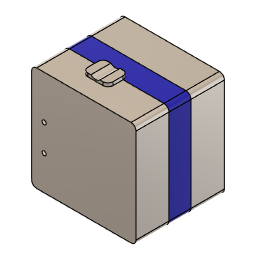
OpenBCI_ESP v18 (Autodesk Fusion 360 design; units mm, degrees)
Autodesk Fusion 360 part; units mm, degrees
sketch "Sketch1" plane through (0, 0, 0) normal (0, 0, 1) x (1, 0, 0)
  line L0 (0, 0) -> (62.5, 0)
  line L1 (62.5, 0) -> (62.5, 62.5)
  line L2 (62.5, 62.5) -> (0, 62.5)
  line L3 (0, 62.5) -> (0, 0)
  line L4 (60, 53.4185) -> (60.5, 53.4185)
  line L5 (60, 6.9185) -> (60.5, 6.9185)
  line L6 (2.5, 53.4185) -> (2, 53.4185)
  circle A0 centre (4.5, 58) radius 1.1
  circle A1 centre (58, 58) radius 1.1
  circle A2 centre (58, 4.5) radius 1.1
  circle A3 centre (4.5, 4.5) radius 1.1
  line L7 (0, 55.25) -> (62.5, 55.25)
  line L8 (0, 7.25) -> (62.5, 7.25)
  line L9 (1.75, 55.25) -> (1.75, 7.25)
  line L10 (60.75, 55.25) -> (60.75, 7.25)
  line L11 (7, 55.25) -> (55.5, 55.25)
  line L12 (55.5, 55.25) -> (55.5, 60)
  line L13 (55.5, 60) -> (7, 60)
  line L14 (7, 60) -> (7, 55.25)
  line L15 (7, 7.25) -> (55.5, 7.25)
  line L16 (55.5, 7.25) -> (55.5, 2.5)
  line L17 (55.5, 2.5) -> (7, 2.5)
  line L18 (7, 2.5) -> (7, 7.25)
  line L19 (10, 60) -> (13.3303, 60)
  line L20 (13.3303, 60) -> (13.3303, 56.25)
  line L21 (13.3303, 56.25) -> (10, 56.25)
  line L22 (10, 56.25) -> (10, 60)
  line L23 (10, 7.25) -> (13.75, 7.25)
  line L24 (13.75, 7.25) -> (13.75, 2.5)
  line L25 (13.75, 2.5) -> (10, 2.5)
  line L26 (10, 2.5) -> (10, 7.25)
  line L27 (40.75, 60) -> (44.5, 60)
  line L28 (44.5, 60) -> (44.5, 56.25)
  line L29 (44.5, 56.25) -> (40.75, 56.25)
  line L30 (40.75, 56.25) -> (40.75, 60)
  line L31 (40.75, 7.25) -> (44.5, 7.25)
  line L32 (44.5, 7.25) -> (44.5, 2.5)
  line L33 (44.5, 2.5) -> (40.75, 2.5)
  line L34 (40.75, 2.5) -> (40.75, 7.25)
  circle A4 centre (4.5, 58) radius 1.9
  circle A5 centre (58, 58) radius 1.9
  circle A6 centre (4.5, 4.5) radius 1.9
  circle A7 centre (58, 4.5) radius 1.9
  line L35 (10, 6.25) -> (13.75, 6.25)
  line L36 (40.75, 6.25) -> (44.5, 6.25)
  dimension "d1" = 62.5
  dimension "d2" = 62.5
  dimension "d5" = 57.5
  dimension "d8" = 2.2
  dimension "d9" = 4.5
  dimension "d10" = 4.5
  dimension "d11" = 2.2
  dimension "d12" = 4.5
  dimension "d13" = 4.5
  dimension "d14" = 2.2
  dimension "d15" = 4.5
  dimension "d16" = 4.5
  dimension "d17" = 2.2
  dimension "d18" = 4.5
  dimension "d19" = 4.5
  dimension "d25" = 7.25
  dimension "d26" = 7.25
  dimension "d27" = 48
  dimension "d28" = 1.75
  dimension "d29" = 1.75
  dimension "d30" = 59
  dimension "d34" = 2.5
  dimension "d35" = 7
  dimension "d36" = 7
  dimension "d37" = 7
  dimension "d38" = 7
  dimension "d39" = 2.5
  dimension "d201" = 3.75
  dimension "d202" = 10
  dimension "d203" = 3.75
  dimension "d204" = 10
  dimension "d205" = 3.75
  dimension "d206" = 18
  dimension "d207" = 3.75
  dimension "d208" = 18
  dimension "d215" = 3.8
  dimension "d216" = 3.8
  dimension "d217" = 3.8
  dimension "d218" = 3.8
  dimension "d219" = 3.75
  dimension "d220" = 3.75
  constraint horizontal L0
  constraint vertical L1
  constraint horizontal L2
  constraint vertical L3
  constraint coincident L0.start L3.end
  constraint coincident L3 L7.start
  constraint coincident L1 L7.end
  constraint perpendicular L1 L7
  constraint coincident L3 L8.start
  constraint coincident L1 L8.end
  constraint perpendicular L1 L8
  constraint coincident L7 L9.start
  constraint coincident L8 L9.end
  constraint perpendicular L8 L9
  constraint coincident L7 L10.start
  constraint coincident L8 L10.end
  constraint perpendicular L8 L10
  constraint horizontal L11
  constraint vertical L12
  constraint horizontal L13
  constraint vertical L14
  constraint coincident L7 L11.start
  constraint horizontal L15
  constraint vertical L16
  constraint horizontal L17
  constraint vertical L18
  constraint coincident L8 L15.start
  constraint horizontal L19
  constraint vertical L20
  constraint horizontal L21
  constraint vertical L22
  constraint coincident L13 L19.start
  constraint horizontal L23
  constraint vertical L24
  constraint horizontal L25
  constraint vertical L26
  constraint coincident L15 L23.start
  constraint horizontal L27
  constraint vertical L28
  constraint horizontal L29
  constraint vertical L30
  constraint coincident L13 L27.start
  constraint horizontal L31
  constraint vertical L32
  constraint horizontal L33
  constraint vertical L34
  constraint coincident L8 L31.start
  constraint concentric A0 A4
  constraint concentric A1 A5
  constraint concentric A3 A6
  constraint concentric A2 A7
  constraint coincident L26 L35.start
  constraint coincident L24 L35.end
  constraint perpendicular L24 L35
  constraint coincident L34 L36.start
  constraint coincident L32 L36.end
  constraint perpendicular L32 L36
  measures "d1" distance of L0.start L0.end
  measures "d2" distance of L0.start L2.end
  measures "d5" distance of L6.start L4.start
  measures "d8" diameter of A0
  measures "d9" distance of L3 A0.centre
  measures "d10" distance of L2 A0.centre
  measures "d11" diameter of A1
  measures "d12" distance of L1 A1.centre
  measures "d13" distance of L2 A1.centre
  measures "d14" diameter of A2
  measures "d15" distance of L1 A2.centre
  measures "d16" distance of L0 A2.centre
  measures "d17" diameter of A3
  measures "d18" distance of L3 A3.centre
  measures "d19" distance of L0 A3.centre
  measures "d25" distance of L2 L7
  measures "d26" distance of L0 L8
  measures "d27" distance of L7 L8
  measures "d28" distance of L1 L10
  measures "d29" distance of L3 L9
  measures "d30" distance of L9 L10
  measures "d34" distance of L2 L13
  measures "d35" distance of L1 L12
  measures "d36" distance of L3 L14
  measures "d37" distance of L1 L16
  measures "d38" distance of L3 L18
  measures "d39" distance of L0 L17
  measures "d201" distance of L19.start L21.end
  measures "d202" distance of L3 L22
  measures "d203" distance of L23.start L23.end
  measures "d204" distance of L3 L26
  measures "d205" distance of L27.start L27.end
  measures "d206" distance of L1 L28
  measures "d207" distance of L31.start L31.end
  measures "d208" distance of L1 L32
  measures "d215" diameter of A4
  measures "d216" diameter of A5
  measures "d217" diameter of A6
  measures "d218" diameter of A7
  measures "d219" distance of L17 L35
  measures "d220" distance of L17 L36
extrude "Extrude1" add sketch "Sketch1" along normal blind 2 contours L0 L1 L3 L8 L16 L17 L18 L25 L33 | L3 L7 L8 L9 | L1 L7 L8 L10 | L1 L2 L3 L7 L12 L13 L14 L19 L27 | L7 L8 L9 L10 L11 L15 L23 L31 | L8 L15 L17 L18 L26 | L8 L15 L16 L17 L32 | L7 L11 L12 L13 L14 L20 L21 L22 L28 L29 L30 | L8 L15 L23 L24 L26 L35 | L8 L15 L31 L32 L34 L36 | L8 L15 L17 L24 L34 | L17 L24 L25 L26 L35 | L17 L32 L33 L34 L36 | L13 L19 L20 L21 L22 | L13 L27 L28 L29 L30 | A4 | A5 | A6 | A7 makes body 1
extrude "Extrude2" add sketch "Sketch1" along normal blind 20 contours L0 L1 L3 L8 L16 L17 L18 L25 L33 | L3 L7 L8 L9 | L1 L7 L8 L10 | L1 L2 L3 L7 L12 L13 L14 L19 L27 | A4 | A5 | A6 | A7 bodies 1
extrude "Extrude18" add sketch "Sketch1" along normal blind 10 from surface at 15 contours L17 L24 L25 L26 L35 | L17 L32 L33 L34 L36 | L13 L19 L20 L21 L22 | L13 L27 L28 L29 L30 bodies 1
chamfer "Chamfer3" distance 3.5 angle 45 4 edges at (11.6651, 56.25, 15) (42.625, 56.25, 15) (42.625, 6.25, 15) (11.875, 6.25, 15) on bodies 1
fillet "Fillet7" radius 3 4 edges at (0, 62.5, 10) (0, 0, 10) (62.5, 62.5, 10) (62.5, 0, 10) on bodies 1
extrude "Extrude20" cut sketch "Sketch1" along normal blind 9 contours A4 | A5 | A6 | A7 bodies 1
sketch "Sketch2" plane through (0, 0, 20) normal (0, 0, 1) x (1, 0, 0)
  line L0 (0, 0) -> (62.5, 0)
  line L1 (62.5, 0) -> (62.5, 62.5)
  line L2 (62.5, 62.5) -> (0, 62.5)
  line L3 (0, 62.5) -> (0, 0)
  line L4 (2, 56.5) -> (52.5, 56.5)
  line L5 (52.5, 56.5) -> (52.5, 6)
  line L6 (52.5, 6) -> (2, 6)
  line L7 (2, 6) -> (2, 56.5)
  circle A0 centre (6, 52.9441) radius 1.1
  circle A1 centre (48.5, 52.5) radius 1.1
  circle A2 centre (6, 10) radius 1.1
  circle A3 centre (48.5, 10) radius 1.1
  line L8 (2, 56.5) -> (10, 56.5)
  line L9 (10, 56.5) -> (10, 48.5)
  line L10 (10, 48.5) -> (2, 48.5)
  line L11 (2, 48.5) -> (2, 56.5)
  line L12 (2, 6) -> (10, 6)
  line L13 (10, 6) -> (10, 14)
  line L14 (10, 14) -> (2, 14)
  line L15 (2, 14) -> (2, 6)
  line L16 (52.5, 6) -> (44.5, 6)
  line L17 (44.5, 6) -> (44.5, 14)
  line L18 (44.5, 14) -> (52.5, 14)
  line L19 (52.5, 14) -> (52.5, 6)
  line L20 (52.5, 56.5) -> (44.5, 56.5)
  line L21 (44.5, 56.5) -> (44.5, 48.5)
  line L22 (44.5, 48.5) -> (52.5, 48.5)
  line L23 (52.5, 48.5) -> (52.5, 56.5)
  line L24 (2, 46.25) -> (0, 46.25)
  line L25 (2, 16.25) -> (0, 16.25)
  line L26 (52.5, 48.5) -> (59.5, 48.5)
  line L27 (59.5, 48.5) -> (59.5, 14)
  line L28 (59.5, 14) -> (52.5, 14)
  line L29 (52.5, 14) -> (52.5, 48.5)
  line L30 (10, 6) -> (44.5, 6)
  line L31 (44.5, 6) -> (44.5, 2.5)
  line L32 (44.5, 2.5) -> (10, 2.5)
  line L33 (10, 2.5) -> (10, 6)
  line L34 (10, 56.5) -> (44.5, 56.5)
  line L35 (44.5, 56.5) -> (44.5, 60)
  line L36 (44.5, 60) -> (10, 60)
  line L37 (10, 60) -> (10, 56.5)
  circle A4 centre (6, 52.9441) radius 0.9
  circle A5 centre (48.5, 52.5) radius 0.9
  circle A6 centre (48.5, 10) radius 0.9
  circle A7 centre (6, 10) radius 0.9
  circle A8 centre (7.5, 36.5) radius 1.25
  circle A9 centre (7.5, 20.5) radius 1.25
  circle A10 centre (18, 36.5) radius 1.25
  circle A11 centre (4.5, 58) radius 0.9
  circle A12 centre (4.5, 4.5) radius 0.9
  circle A13 centre (58, 4.5) radius 0.9
  circle A14 centre (58, 58) radius 0.9
  line L38 (44.5, 60) -> (39.5, 60)
  line L39 (39.5, 56.5) -> (44.5, 56.5)
  line L40 (44.5, 56.5) -> (44.5, 60)
  line L41 (10, 60) -> (15, 60)
  line L42 (15, 60) -> (15, 56.5)
  line L43 (15, 56.5) -> (10, 56.5)
  line L44 (10, 56.5) -> (10, 60)
  line L45 (44.5, 2.5) -> (39.5, 2.5)
  line L46 (39.5, 6) -> (44.5, 6)
  line L47 (44.5, 6) -> (44.5, 2.5)
  line L48 (10, 2.5) -> (15, 2.5)
  line L49 (15, 2.5) -> (15, 6)
  line L50 (15, 6) -> (10, 6)
  line L51 (10, 6) -> (10, 2.5)
  line L52 (59.5, 48.5) -> (56, 48.5)
  line L53 (56, 48.5) -> (56, 43.5)
  line L54 (56, 43.5) -> (59.5, 43.5)
  line L55 (59.5, 43.5) -> (59.5, 48.5)
  line L56 (59.5, 14) -> (56, 14)
  line L57 (56, 14) -> (56, 19)
  line L58 (56, 19) -> (59.5, 19)
  line L59 (59.5, 19) -> (59.5, 14)
  dimension "d42" = 62.5
  dimension "d43" = 62.5
  dimension "d44" = 50.5
  dimension "d45" = 50.5
  dimension "d46" = 6
  dimension "d47" = 2
  dimension "d48" = 2.2
  dimension "d49" = 4
  dimension "d50" = 2.2
  dimension "d51" = 4
  dimension "d52" = 4
  dimension "d53" = 2.2
  dimension "d54" = 2.2
  dimension "d55" = 4
  dimension "d56" = 4
  dimension "d57" = 4
  dimension "d58" = 4
  dimension "d59" = 8
  dimension "d60" = 8
  dimension "d61" = 8
  dimension "d62" = 8
  dimension "d63" = 8
  dimension "d64" = 8
  dimension "d65" = 8
  dimension "d66" = 8
  dimension "d67" = 30
  dimension "d68" = 10.25
  dimension "d69" = 7
  dimension "d70" = 3.5
  dimension "d71" = 3.5
  dimension "d105" = 1.8
  dimension "d106" = 1.8
  dimension "d107" = 1.8
  dimension "d108" = 1.8
  dimension "d109" = 2.5
  dimension "d110" = 2.5
  dimension "d111" = 2.5
  dimension "d112" = 5.5
  dimension "d113" = 5.5
  dimension "d114" = 14.5
  dimension "d115" = 20
  dimension "d116" = 20
  dimension "d117" = 16
  dimension "d133" = 1.8
  dimension "d135" = 1.8
  dimension "d136" = 1.8
  dimension "d137" = 4.5
  dimension "d138" = 4.5
  dimension "d139" = 4.5
  dimension "d140" = 4.5
  dimension "d141" = 4.5
  dimension "d142" = 4.5
  dimension "d145" = 1.8
  dimension "d146" = 4.5
  dimension "d147" = 4.5
  dimension "d176" = 16
  dimension "d189" = 3.5
  dimension "d190" = 5
  dimension "d191" = 3.5
  dimension "d193" = 3.5
  dimension "d194" = 5
  dimension "d195" = 3.5
  dimension "d223" = 3.5
  dimension "d224" = 5
  dimension "d225" = 3.5
  dimension "d226" = 5
  constraint horizontal L0
  constraint vertical L1
  constraint horizontal L2
  constraint vertical L3
  constraint coincident L0.start L3.end
  constraint horizontal L4
  constraint vertical L5
  constraint horizontal L6
  constraint vertical L7
  constraint horizontal L8
  constraint vertical L9
  constraint horizontal L10
  constraint vertical L11
  constraint horizontal L12
  constraint vertical L13
  constraint horizontal L14
  constraint vertical L15
  constraint horizontal L16
  constraint vertical L17
  constraint horizontal L18
  constraint vertical L19
  constraint horizontal L20
  constraint vertical L21
  constraint horizontal L22
  constraint vertical L23
  constraint coincident L7 L24.start
  constraint coincident L3 L24.end
  constraint perpendicular L3 L24
  constraint coincident L7 L25.start
  constraint coincident L3 L25.end
  constraint perpendicular L7 L25
  constraint horizontal L26
  constraint vertical L27
  constraint horizontal L28
  constraint vertical L29
  constraint horizontal L30
  constraint vertical L31
  constraint horizontal L32
  constraint vertical L33
  constraint horizontal L34
  constraint vertical L35
  constraint horizontal L36
  constraint vertical L37
  constraint concentric A0 A4
  constraint concentric A1 A5
  constraint concentric A3 A6
  constraint concentric A2 A7
  constraint horizontal L38
  constraint horizontal L39
  constraint vertical L40
  constraint horizontal L41
  constraint vertical L42
  constraint horizontal L43
  constraint vertical L44
  constraint horizontal L45
  constraint horizontal L46
  constraint vertical L47
  constraint horizontal L48
  constraint vertical L49
  constraint horizontal L50
  constraint vertical L51
  constraint horizontal L52
  constraint vertical L53
  constraint horizontal L54
  constraint vertical L55
  constraint horizontal L56
  constraint vertical L57
  constraint horizontal L58
  constraint vertical L59
  measures "d42" distance of L1 L3
  measures "d43" distance of L0 L2
  measures "d44" distance of L4.start L4.end
  measures "d45" distance of L4.start L6.end
  measures "d46" distance of L2 L4
  measures "d47" distance of L3 L7
  measures "d48" diameter of A0
  measures "d49" distance of L7 A0.centre
  measures "d50" diameter of A1
  measures "d51" distance of L5 A1.centre
  measures "d52" distance of L4 A1.centre
  measures "d53" diameter of A2
  measures "d54" diameter of A3
  measures "d55" distance of L5 A3.centre
  measures "d56" distance of L6 A3.centre
  measures "d57" distance of L6 A2.centre
  measures "d58" distance of L7 A2.centre
  measures "d59" distance of L4.start L8.end
  measures "d60" distance of L4.start L10.end
  measures "d61" distance of L6.end L12.end
  measures "d62" distance of L6.end L14.end
  measures "d63" distance of L5.end L16.end
  measures "d64" distance of L5.end L18.end
  measures "d65" distance of L4.end L20.end
  measures "d66" distance of L4.end L22.end
  measures "d67" distance of L24 L25
  measures "d68" distance of L12 L25
  measures "d69" distance of L22.end L26.end
  measures "d70" distance of L12.end L32.end
  measures "d71" distance of L8.end L36.end
  measures "d105" diameter of A4
  measures "d106" diameter of A5
  measures "d107" diameter of A6
  measures "d108" diameter of A7
  measures "d109" diameter of A8
  measures "d110" diameter of A9
  measures "d111" diameter of A10
  measures "d112" distance of L7 A8.centre
  measures "d113" distance of L7 A9.centre
  measures "d114" distance of L30 A9.centre
  measures "d115" distance of L34 A8.centre
  measures "d116" distance of L4 A10.centre
  measures "d117" distance of L7 A10.centre
  measures "d133" diameter of A11
  measures "d135" diameter of A12
  measures "d136" diameter of A13
  measures "d137" distance of L1 A13.centre
  measures "d138" distance of L0 A13.centre
  measures "d139" distance of L3 A12.centre
  measures "d140" distance of L0 A12.centre
  measures "d141" distance of L3 A11.centre
  measures "d142" distance of L2 A11.centre
  measures "d145" diameter of A14
  measures "d146" distance of L2 A14.centre
  measures "d147" distance of L1 A14.centre
  measures "d176" distance of A8.centre A9.centre
  measures "d189" distance of L35.end L20.end
  measures "d190" distance of L36.end L41.end
  measures "d191" distance of L36.end L8.end
  measures "d193" distance of L31.end L16.end
  measures "d194" distance of L32.end L48.end
  measures "d195" distance of L32.end L12.end
  measures "d223" distance of L26.end L52.end
  measures "d224" distance of L26.end L54.end
  measures "d225" distance of L27.end L56.end
  measures "d226" distance of L27.end L58.end
extrude "Extrude3" add sketch "Sketch2" along normal blind 2 separate body contours L0 L1 L2 L3 L4 L5 L6 L7 L8 L11 L12 L15 L16 L19 L20 L23 L24 L25 L26 L27 L28 L31 L32 L33 L35 L36 L37 L38 L40 L41 L44 L45 L47 L48 L51 L52 L55 L56 L59 makes body 2
extrude "Extrude4" add sketch "Sketch2" along normal blind 11.2 from surface at 2 contours L0 L1 L2 L3 L4 L5 L6 L7 L8 L11 L12 L15 L16 L19 L20 L23 L24 L25 L26 L27 L28 L31 L32 L33 L35 L36 L37 L38 L40 L41 L44 L45 L47 L48 L51 L52 L55 L56 L59 | L6 L7 L12 L13 L14 L15 | L4 L7 L8 L9 L10 L11 | L5 L6 L16 L17 L18 L19 | L4 L5 L20 L21 L22 L23 | A0 | A1 | A2 | A3 bodies 2
extrude "Extrude5" add sketch "Sketch2" along normal blind 4.2 from surface at 9 contours L3 L7 L24 L25 bodies 2
fillet "Fillet3" radius 3 4 edges at (0, 62.5, 26.6) (62.5, 62.5, 26.6) (0, 0, 26.6) (62.5, 0, 26.6) on bodies 2
extrude "Extrude6" add sketch "Sketch2" along normal blind 1.2 from surface at 13.2 separate body contours L0 L1 L2 L3 L4 L5 L6 L7 L8 L11 L12 L15 L16 L19 L20 L23 L24 L25 L26 L27 L28 L31 L32 L33 L35 L36 L37 L38 L40 L41 L44 L45 L47 L48 L51 L52 L55 L56 L59 | L3 L7 L24 L25 | A11 | A12 | A13 | A14 makes body 3
extrude "Extrude7" add sketch "Sketch2" along normal blind 16.5 from surface at 14.4 contours L0 L1 L2 L3 L4 L5 L6 L7 L8 L11 L12 L15 L16 L19 L20 L23 L24 L25 L26 L27 L28 L31 L32 L33 L35 L36 L37 L38 L40 L41 L44 L45 L47 L48 L51 L52 L55 L56 L59 | L3 L7 L24 L25 | L6 L7 L12 L13 L14 L15 | L4 L7 L8 L9 L10 L11 | L5 L6 L16 L17 L18 L19 | L4 L5 L20 L21 L22 L23 | A0 | A1 | A2 | A3 | A11 | A12 | A13 | A14 bodies 3
extrude "Extrude8" add sketch "Sketch2" along normal blind 1 from surface at 30.9 contours L0 L1 L2 L3 L4 L5 L6 L7 L8 L11 L12 L15 L16 L19 L20 L23 L24 L25 L26 L27 L28 L31 L32 L33 L35 L36 L37 L38 L40 L41 L44 L45 L47 L48 L51 L52 L55 L56 L59 | L3 L7 L24 L25 | L4 L5 L6 L7 L9 L10 L13 L14 L17 L18 L21 L22 L29 L30 L34 L39 L43 L46 L50 | L6 L7 L12 L13 L14 L15 | L4 L7 L8 L9 L10 L11 | L6 L30 L32 L33 L48 L49 L50 L51 | L4 L34 L36 L37 L41 L42 L43 L44 | L6 L30 L31 L32 L45 L46 L47 L49 | L4 L34 L35 L36 L38 L39 L40 L42 | L5 L6 L16 L17 L18 L19 | L4 L5 L20 L21 L22 L23 | L5 L26 L27 L28 L29 L53 L54 L57 L58 | L27 L28 L56 L57 L58 L59 | L26 L27 L52 L53 L54 L55 | A0 | A1 | A2 | A3 | A4 | A5 | A6 | A7 | A11 | A12 | A13 | A14 bodies 3
extrude "Extrude10" add sketch "Sketch2" along normal blind 1 from surface at 31.9 contours L0 L1 L2 L3 L4 L5 L6 L7 L8 L11 L12 L15 L16 L19 L20 L23 L24 L25 L26 L27 L28 L31 L32 L33 L35 L36 L37 L38 L40 L41 L44 L45 L47 L48 L51 L52 L55 L56 L59 | L3 L7 L24 L25 | L4 L5 L6 L7 L9 L10 L13 L14 L17 L18 L21 L22 L29 L30 L34 L39 L43 L46 L50 | L6 L7 L12 L13 L14 L15 | L4 L7 L8 L9 L10 L11 | L6 L30 L32 L33 L48 L49 L50 L51 | L4 L34 L36 L37 L41 L42 L43 L44 | L6 L30 L31 L32 L45 L46 L47 L49 | L4 L34 L35 L36 L38 L39 L40 L42 | L5 L6 L16 L17 L18 L19 | L4 L5 L20 L21 L22 L23 | L5 L26 L27 L28 L29 L53 L54 L57 L58 | L27 L28 L56 L57 L58 L59 | L26 L27 L52 L53 L54 L55 | A0 | A1 | A2 | A3 | A4 | A5 | A6 | A7 | A10 | A11 | A12 | A13 | A14 bodies 3
fillet "Fillet4" radius 3 4 edges at (0, 0, 42.55) (62.5, 0, 42.55) (0, 62.5, 42.55) (62.5, 62.5, 42.55) on bodies 3
sketch "Sketch4" plane through (0, 0, 0) normal (-1, 0, 0) x (0, 0, 1)
  line L0 (33.2, 35.5) -> (37.2, 35.5)
  line L1 (37.2, 35.5) -> (37.2, 20.5)
  line L2 (37.2, 20.5) -> (33.2, 20.5)
  line L3 (33.2, 20.5) -> (33.2, 35.5)
  line L4 (33.2, 59.5) -> (52.9, 59.5)
  line L5 (45.2, 33.5) -> (51.2, 33.5)
  line L6 (51.2, 33.5) -> (51.2, 22.5)
  line L7 (51.2, 22.5) -> (45.2, 22.5)
  line L8 (45.2, 22.5) -> (45.2, 33.5)
  line L9 (20, 62.5) -> (20, 0)
  dimension "d95" = 4
  dimension "d96" = 15
  dimension "d97" = 24
  dimension "d98" = 6
  dimension "d99" = 11
  dimension "d100" = 13.2
  dimension "d101" = 12
  dimension "d102" = 26
  constraint horizontal L0
  constraint vertical L1
  constraint horizontal L2
  constraint vertical L3
  constraint horizontal L5
  constraint vertical L6
  constraint horizontal L7
  constraint vertical L8
  measures "d95" distance of L0.start L0.end
  measures "d96" distance of L0.start L2.end
  measures "d97" distance of L0 L4
  measures "d98" distance of L5.start L5.end
  measures "d99" distance of L5.start L7.end
  measures "d100" distance of L3 L9
  measures "d101" distance of L3 L8
  measures "d102" distance of L4 L5
extrude "Extrude9" cut sketch "Sketch4" against normal blind 2 bodies 3
sketch "Sketch6" plane through (0, 62.5, 0) normal (0, 1, 0) x (-1, 0, 0)
  line L0 (-24, 33.2) -> (-34, 33.2)
  line L1 (-34, 33.2) -> (-34, 39.2)
  line L2 (-34, 39.2) -> (-24, 39.2)
  line L3 (-24, 39.2) -> (-24, 33.2)
  line L4 (-62.5, 20) -> (0, 20)
  line L5 (0, 33.2) -> (0, 37.2)
  line L6 (-3, 52.9) -> (-59.5, 52.9)
  dimension "d148" = 10
  dimension "d149" = 6
  dimension "d150" = 13.2
  dimension "d151" = 24
  dimension "d230" = 13.7
  constraint horizontal L0
  constraint vertical L1
  constraint horizontal L2
  constraint vertical L3
  measures "d148" distance of L0.start L0.end
  measures "d149" distance of L0.start L2.end
  measures "d150" distance of L0 L4
  measures "d151" distance of L3 L5
  measures "d230" distance of L2 L6
extrude "Extrude12" cut sketch "Sketch6" against normal blind 2.5 bodies 3
sketch "Sketch7" plane through (0, 62.5, 0) normal (0, 1, 0) x (-1, 0, 0)
  line L0 (-24, 33.2078) -> (-31, 33.2078)
  line L1 (-31, 33.2078) -> (-31, 39.2078)
  line L2 (-31, 39.2078) -> (-24, 39.2078)
  line L3 (-24, 39.2078) -> (-24, 33.2078)
  line L4 (-20, 30.2) -> (-35, 30.2)
  line L5 (-35, 30.2) -> (-35, 42.2)
  line L6 (-35, 42.2) -> (-20, 42.2)
  line L7 (-20, 42.2) -> (-20, 30.2)
  line L8 (-28.556, 37.7078) -> (-26.556, 37.7078)
  line L9 (-26.556, 37.7078) -> (-26.556, 35.7078)
  line L10 (-26.556, 35.7078) -> (-28.556, 35.7078)
  line L11 (-28.556, 35.7078) -> (-28.556, 37.7078)
  line L12 (0, 52.9) -> (0, 33.2)
  line L13 (-3, 52.9) -> (-59.5, 52.9)
  line L14 (-34, 39.2) -> (-24, 39.2)
  dimension "d154" = 7
  dimension "d155" = 6
  dimension "d156" = 15
  dimension "d157" = 12
  dimension "d158" = 4
  dimension "d160" = 2
  dimension "d161" = 2
  dimension "d227" = 2.5
  dimension "d228" = 20
  dimension "d229" = 13.7
  constraint horizontal L0
  constraint vertical L1
  constraint horizontal L2
  constraint vertical L3
  constraint horizontal L4
  constraint vertical L5
  constraint horizontal L6
  constraint vertical L7
  constraint horizontal L8
  constraint vertical L9
  constraint horizontal L10
  constraint vertical L11
  measures "d154" distance of L0.start L0.end
  measures "d155" distance of L0.start L2.end
  measures "d156" distance of L4.start L4.end
  measures "d157" distance of L4.start L6.end
  measures "d158" distance of L3 L7
  measures "d160" distance of L8.start L8.end
  measures "d161" distance of L8.start L10.end
  measures "d227" distance of L0 L10
  measures "d228" distance of L7 L12
  measures "d229" distance of L13 L14
extrude "Extrude13" add sketch "Sketch7" along normal blind 2 separate body contours L0 L1 L3 L14 | L1 L2 L3 L14 | L4 L5 L6 L7 | L8 L9 L10 L11 makes body 4
extrude "Extrude14" add sketch "Sketch7" against normal blind 2.7 contours L0 L1 L3 L14 | L1 L2 L3 L14 | L8 L9 L10 L11 bodies 4
extrude "Extrude15" add sketch "Sketch7" against normal blind 2 from surface at -2.7 contours L0 L1 L3 L14 | L1 L2 L3 L14 | L4 L5 L6 L7 bodies 4
extrude "Extrude16" add sketch "Sketch7" against normal blind 0.8 from surface at -4.7 contours L0 L1 L3 L14 | L1 L2 L3 L14 bodies 4
extrude "Extrude17" add sketch "Sketch2" along normal blind 12 from surface at 10 contours L6 L30 L32 L33 L48 L49 L50 L51 | L4 L34 L36 L37 L41 L42 L43 L44 | L27 L28 L56 L57 L58 L59 | L26 L27 L52 L53 L54 L55 bodies 3
chamfer "Chamfer2" distance 3.5 angle 45 4 edges at (12.5, 56.5, 42) (12.5, 6, 42) (56, 16.5, 42) (56, 46, 42) on bodies 3
fillet "Fillet8" radius 3 4 edges at (35, 63.5, 30.2) (35, 63.5, 42.2) (20, 63.5, 42.2) (20, 63.5, 30.2) on bodies 4
sketch "Sketch8" plane through (0, 0, 42.2) normal (0, 0, 1) x (1, 0, 0)
  circle A0 centre (27.4814, 67.3123) radius 3.9076
extrude "Extrude19" cut sketch "Sketch8" against normal blind 12 bodies 4
named bodies: "Battery", "Input_8", "Base", "Switch"
